Autodesk Fusion 360 part; units mm, degrees
note: some values were not read from the file. Set by a fixed rule: which face or edge a step refers to.
(part 3 of 4)
sketch "Sketch2 (4)" plane through (0, 0, 58.4) normal (0, 0, -1) x (1, 0, 0) in component "M5xxx-lid"
  line L0 (-91.022, 50.6335) -> (-91.022, 57.5617)
  line L1 (-91.022, 57.5617) -> (-97.022, 61.0258)
  line L2 (-97.022, 61.0258) -> (-103.022, 57.5617)
  line L3 (-103.022, 57.5617) -> (-103.022, 50.6335)
  line L4 (-103.022, 50.6335) -> (-97.022, 47.1694)
  line L5 (-97.022, 47.1694) -> (-91.022, 50.6335)
  line L6 (-96.022, 38.6335) -> (-90.022, 35.1694)
  line L7 (-90.022, 35.1694) -> (-84.022, 38.6335)
  line L8 (-96.022, 45.5617) -> (-96.022, 38.6335)
  line L9 (-84.022, 38.6335) -> (-84.022, 45.5617)
  line L10 (-90.022, 49.0258) -> (-96.022, 45.5617)
  line L11 (-84.022, 45.5617) -> (-90.022, 49.0258)
  line L12 (-82.022, 38.6335) -> (-76.022, 35.1694)
  line L13 (-82.022, 45.5617) -> (-82.022, 38.6335)
  line L14 (-70.022, 45.5617) -> (-76.022, 49.0258)
  line L15 (-76.022, 49.0258) -> (-82.022, 45.5617)
  line L16 (-76.022, 35.1694) -> (-70.022, 38.6335)
  line L17 (-83.022, 61.0258) -> (-89.022, 57.5617)
  line L18 (-77.022, 57.5617) -> (-83.022, 61.0258)
  line L19 (-70.022, 38.6335) -> (-70.022, 45.5617)
  line L20 (-83.022, 47.1694) -> (-77.022, 50.6335)
  line L21 (-89.022, 50.6335) -> (-83.022, 47.1694)
  line L22 (-89.022, 57.5617) -> (-89.022, 50.6335)
  line L23 (-77.022, 50.6335) -> (-77.022, 57.5617)
  line L24 (-68.022, 38.6335) -> (-62.022, 35.1694)
  line L25 (-68.022, 45.5617) -> (-68.022, 38.6335)
  line L26 (-56.022, 45.5617) -> (-62.022, 49.0258)
  line L27 (-62.022, 49.0258) -> (-68.022, 45.5617)
  line L28 (-62.022, 35.1694) -> (-56.022, 38.6335)
  line L29 (-69.022, 61.0258) -> (-75.022, 57.5617)
  line L30 (-63.022, 57.5617) -> (-69.022, 61.0258)
  line L31 (-56.022, 38.6335) -> (-56.022, 45.5617)
  line L32 (-69.022, 47.1694) -> (-63.022, 50.6335)
  line L33 (-75.022, 50.6335) -> (-69.022, 47.1694)
  line L34 (-75.022, 57.5617) -> (-75.022, 50.6335)
  line L35 (-63.022, 50.6335) -> (-63.022, 57.5617)
  line L36 (-54.022, 38.6335) -> (-48.022, 35.1694)
  line L37 (-54.022, 45.5617) -> (-54.022, 38.6335)
  line L38 (-42.022, 45.5617) -> (-48.022, 49.0258)
  line L39 (-48.022, 49.0258) -> (-54.022, 45.5617)
  line L40 (-48.022, 35.1694) -> (-42.022, 38.6335)
  line L41 (-55.022, 61.0258) -> (-61.022, 57.5617)
  line L42 (-49.022, 57.5617) -> (-55.022, 61.0258)
  line L43 (-42.022, 38.6335) -> (-42.022, 45.5617)
  line L44 (-55.022, 47.1694) -> (-49.022, 50.6335)
  line L45 (-61.022, 50.6335) -> (-55.022, 47.1694)
  line L46 (-61.022, 57.5617) -> (-61.022, 50.6335)
  line L47 (-49.022, 50.6335) -> (-49.022, 57.5617)
  line L48 (-40.022, 38.6335) -> (-34.022, 35.1694)
  line L49 (-40.022, 45.5617) -> (-40.022, 38.6335)
  line L50 (-28.022, 45.5617) -> (-34.022, 49.0258)
  line L51 (-34.022, 49.0258) -> (-40.022, 45.5617)
  line L52 (-34.022, 35.1694) -> (-28.022, 38.6335)
  line L53 (-41.022, 61.0258) -> (-47.022, 57.5617)
  line L54 (-35.022, 57.5617) -> (-41.022, 61.0258)
  line L55 (-28.022, 38.6335) -> (-28.022, 45.5617)
  line L56 (-41.022, 47.1694) -> (-35.022, 50.6335)
  line L57 (-47.022, 50.6335) -> (-41.022, 47.1694)
  line L58 (-47.022, 57.5617) -> (-47.022, 50.6335)
  line L59 (-35.022, 50.6335) -> (-35.022, 57.5617)
  line L60 (-26.022, 38.6335) -> (-20.022, 35.1694)
  line L61 (-26.022, 45.5617) -> (-26.022, 38.6335)
  line L62 (-14.022, 45.5617) -> (-20.022, 49.0258)
  line L63 (-20.022, 49.0258) -> (-26.022, 45.5617)
  line L64 (-20.022, 35.1694) -> (-14.022, 38.6335)
  line L65 (-27.022, 61.0258) -> (-33.022, 57.5617)
  line L66 (-21.022, 57.5617) -> (-27.022, 61.0258)
  line L67 (-14.022, 38.6335) -> (-14.022, 45.5617)
  line L68 (-27.022, 47.1694) -> (-21.022, 50.6335)
  line L69 (-33.022, 50.6335) -> (-27.022, 47.1694)
  line L70 (-33.022, 57.5617) -> (-33.022, 50.6335)
  line L71 (-21.022, 50.6335) -> (-21.022, 57.5617)
  line L72 (-12.022, 38.6335) -> (-6.022, 35.1694)
  line L73 (-12.022, 45.5617) -> (-12.022, 38.6335)
  line L74 (-0.022, 45.5617) -> (-6.022, 49.0258)
  line L75 (-6.022, 49.0258) -> (-12.022, 45.5617)
  line L76 (-6.022, 35.1694) -> (-0.022, 38.6335)
  line L77 (-13.022, 61.0258) -> (-19.022, 57.5617)
  line L78 (-7.022, 57.5617) -> (-13.022, 61.0258)
  line L79 (-0.022, 38.6335) -> (-0.022, 45.5617)
  line L80 (-13.022, 47.1694) -> (-7.022, 50.6335)
  line L81 (-19.022, 50.6335) -> (-13.022, 47.1694)
  line L82 (-19.022, 57.5617) -> (-19.022, 50.6335)
  line L83 (-7.022, 50.6335) -> (-7.022, 57.5617)
  line L84 (1.978, 38.6335) -> (7.978, 35.1694)
  line L85 (1.978, 45.5617) -> (1.978, 38.6335)
  line L86 (13.978, 45.5617) -> (7.978, 49.0258)
  line L87 (7.978, 49.0258) -> (1.978, 45.5617)
  line L88 (7.978, 35.1694) -> (13.978, 38.6335)
  line L89 (0.978, 61.0258) -> (-5.022, 57.5617)
  line L90 (6.978, 57.5617) -> (0.978, 61.0258)
  line L91 (13.978, 38.6335) -> (13.978, 45.5617)
  line L92 (0.978, 47.1694) -> (6.978, 50.6335)
  line L93 (-5.022, 50.6335) -> (0.978, 47.1694)
  line L94 (-5.022, 57.5617) -> (-5.022, 50.6335)
  line L95 (6.978, 50.6335) -> (6.978, 57.5617)
  line L96 (15.978, 38.6335) -> (21.978, 35.1694)
  line L97 (15.978, 45.5617) -> (15.978, 38.6335)
  line L98 (27.978, 45.5617) -> (21.978, 49.0258)
  line L99 (21.978, 49.0258) -> (15.978, 45.5617)
  line L100 (21.978, 35.1694) -> (27.978, 38.6335)
  line L101 (14.978, 61.0258) -> (8.978, 57.5617)
  line L102 (20.978, 57.5617) -> (14.978, 61.0258)
  line L103 (27.978, 38.6335) -> (27.978, 45.5617)
  line L104 (14.978, 47.1694) -> (20.978, 50.6335)
  line L105 (8.978, 50.6335) -> (14.978, 47.1694)
  line L106 (8.978, 57.5617) -> (8.978, 50.6335)
  line L107 (20.978, 50.6335) -> (20.978, 57.5617)
  line L108 (29.978, 38.6335) -> (35.978, 35.1694)
  line L109 (29.978, 45.5617) -> (29.978, 38.6335)
  line L110 (41.978, 45.5617) -> (35.978, 49.0258)
  line L111 (35.978, 49.0258) -> (29.978, 45.5617)
  line L112 (35.978, 35.1694) -> (41.978, 38.6335)
  line L113 (28.978, 61.0258) -> (22.978, 57.5617)
  line L114 (34.978, 57.5617) -> (28.978, 61.0258)
  line L115 (41.978, 38.6335) -> (41.978, 45.5617)
  line L116 (28.978, 47.1694) -> (34.978, 50.6335)
  line L117 (22.978, 50.6335) -> (28.978, 47.1694)
  line L118 (22.978, 57.5617) -> (22.978, 50.6335)
  line L119 (34.978, 50.6335) -> (34.978, 57.5617)
  line L120 (43.978, 38.6335) -> (49.978, 35.1694)
  line L121 (43.978, 45.5617) -> (43.978, 38.6335)
  line L122 (55.978, 45.5617) -> (49.978, 49.0258)
  line L123 (49.978, 49.0258) -> (43.978, 45.5617)
  line L124 (49.978, 35.1694) -> (55.978, 38.6335)
  line L125 (42.978, 61.0258) -> (36.978, 57.5617)
  line L126 (48.978, 57.5617) -> (42.978, 61.0258)
  line L127 (55.978, 38.6335) -> (55.978, 45.5617)
  line L128 (42.978, 47.1694) -> (48.978, 50.6335)
  line L129 (36.978, 50.6335) -> (42.978, 47.1694)
  line L130 (36.978, 57.5617) -> (36.978, 50.6335)
  line L131 (48.978, 50.6335) -> (48.978, 57.5617)
  line L132 (57.978, 38.6335) -> (63.978, 35.1694)
  line L133 (57.978, 45.5617) -> (57.978, 38.6335)
  line L134 (69.978, 45.5617) -> (63.978, 49.0258)
  line L135 (63.978, 49.0258) -> (57.978, 45.5617)
  line L136 (63.978, 35.1694) -> (69.978, 38.6335)
  line L137 (56.978, 61.0258) -> (50.978, 57.5617)
  line L138 (62.978, 57.5617) -> (56.978, 61.0258)
  line L139 (69.978, 38.6335) -> (69.978, 45.5617)
  line L140 (56.978, 47.1694) -> (62.978, 50.6335)
  line L141 (50.978, 50.6335) -> (56.978, 47.1694)
  line L142 (50.978, 57.5617) -> (50.978, 50.6335)
  line L143 (62.978, 50.6335) -> (62.978, 57.5617)
  line L144 (71.978, 38.6335) -> (77.978, 35.1694)
  line L145 (71.978, 45.5617) -> (71.978, 38.6335)
  line L146 (83.978, 45.5617) -> (77.978, 49.0258)
  line L147 (77.978, 49.0258) -> (71.978, 45.5617)
  line L148 (77.978, 35.1694) -> (83.978, 38.6335)
  line L149 (70.978, 61.0258) -> (64.978, 57.5617)
  line L150 (76.978, 57.5617) -> (70.978, 61.0258)
  line L151 (83.978, 38.6335) -> (83.978, 45.5617)
  line L152 (70.978, 47.1694) -> (76.978, 50.6335)
  line L153 (64.978, 50.6335) -> (70.978, 47.1694)
  line L154 (64.978, 57.5617) -> (64.978, 50.6335)
  line L155 (76.978, 50.6335) -> (76.978, 57.5617)
  line L156 (85.978, 38.6335) -> (91.978, 35.1694)
  line L157 (85.978, 45.5617) -> (85.978, 38.6335)
  line L158 (97.978, 45.5617) -> (91.978, 49.0258)
  line L159 (91.978, 49.0258) -> (85.978, 45.5617)
  line L160 (91.978, 35.1694) -> (97.978, 38.6335)
  line L161 (84.978, 61.0258) -> (78.978, 57.5617)
  line L162 (90.978, 57.5617) -> (84.978, 61.0258)
  line L163 (97.978, 38.6335) -> (97.978, 45.5617)
  line L164 (84.978, 47.1694) -> (90.978, 50.6335)
  line L165 (78.978, 50.6335) -> (84.978, 47.1694)
  line L166 (78.978, 57.5617) -> (78.978, 50.6335)
  line L167 (90.978, 50.6335) -> (90.978, 57.5617)
  line L168 (-96.022, 14.6335) -> (-90.022, 11.1694)
  line L169 (-96.022, 21.5617) -> (-96.022, 14.6335)
  line L170 (-84.022, 21.5617) -> (-90.022, 25.0258)
  line L171 (-90.022, 25.0258) -> (-96.022, 21.5617)
  line L172 (-90.022, 11.1694) -> (-84.022, 14.6335)
  line L173 (-97.022, 37.0258) -> (-103.022, 33.5617)
  line L174 (-91.022, 33.5617) -> (-97.022, 37.0258)
  line L175 (-84.022, 14.6335) -> (-84.022, 21.5617)
  line L176 (-97.022, 23.1694) -> (-91.022, 26.6335)
  line L177 (-103.022, 26.6335) -> (-97.022, 23.1694)
  line L178 (-103.022, 33.5617) -> (-103.022, 26.6335)
  line L179 (-91.022, 26.6335) -> (-91.022, 33.5617)
  line L180 (-82.022, 14.6335) -> (-76.022, 11.1694)
  line L181 (-82.022, 21.5617) -> (-82.022, 14.6335)
  line L182 (-70.022, 21.5617) -> (-76.022, 25.0258)
  line L183 (-76.022, 25.0258) -> (-82.022, 21.5617)
  line L184 (-76.022, 11.1694) -> (-70.022, 14.6335)
  line L185 (-83.022, 37.0258) -> (-89.022, 33.5617)
  line L186 (-77.022, 33.5617) -> (-83.022, 37.0258)
  line L187 (-70.022, 14.6335) -> (-70.022, 21.5617)
  line L188 (-83.022, 23.1694) -> (-77.022, 26.6335)
  line L189 (-89.022, 26.6335) -> (-83.022, 23.1694)
  line L190 (-89.022, 33.5617) -> (-89.022, 26.6335)
  line L191 (-77.022, 26.6335) -> (-77.022, 33.5617)
  line L192 (-68.022, 14.6335) -> (-62.022, 11.1694)
  line L193 (-68.022, 21.5617) -> (-68.022, 14.6335)
  line L194 (-56.022, 21.5617) -> (-62.022, 25.0258)
  line L195 (-62.022, 25.0258) -> (-68.022, 21.5617)
  line L196 (-62.022, 11.1694) -> (-56.022, 14.6335)
  line L197 (-69.022, 37.0258) -> (-75.022, 33.5617)
  line L198 (-63.022, 33.5617) -> (-69.022, 37.0258)
  line L199 (-56.022, 14.6335) -> (-56.022, 21.5617)
  line L200 (-69.022, 23.1694) -> (-63.022, 26.6335)
  line L201 (-75.022, 26.6335) -> (-69.022, 23.1694)
  line L202 (-75.022, 33.5617) -> (-75.022, 26.6335)
  line L203 (-63.022, 26.6335) -> (-63.022, 33.5617)
  line L204 (-54.022, 14.6335) -> (-48.022, 11.1694)
  line L205 (-54.022, 21.5617) -> (-54.022, 14.6335)
  line L206 (-42.022, 21.5617) -> (-48.022, 25.0258)
  line L207 (-48.022, 25.0258) -> (-54.022, 21.5617)
  line L208 (-48.022, 11.1694) -> (-42.022, 14.6335)
  line L209 (-55.022, 37.0258) -> (-61.022, 33.5617)
  line L210 (-49.022, 33.5617) -> (-55.022, 37.0258)
  line L211 (-42.022, 14.6335) -> (-42.022, 21.5617)
  line L212 (-55.022, 23.1694) -> (-49.022, 26.6335)
  line L213 (-61.022, 26.6335) -> (-55.022, 23.1694)
  line L214 (-61.022, 33.5617) -> (-61.022, 26.6335)
  line L215 (-49.022, 26.6335) -> (-49.022, 33.5617)
  line L216 (-40.022, 14.6335) -> (-34.022, 11.1694)
  line L217 (-40.022, 21.5617) -> (-40.022, 14.6335)
  line L218 (-28.022, 21.5617) -> (-34.022, 25.0258)
  line L219 (-34.022, 25.0258) -> (-40.022, 21.5617)
  line L220 (-34.022, 11.1694) -> (-28.022, 14.6335)
  line L221 (-41.022, 37.0258) -> (-47.022, 33.5617)
  line L222 (-35.022, 33.5617) -> (-41.022, 37.0258)
  line L223 (-28.022, 14.6335) -> (-28.022, 21.5617)
  line L224 (-41.022, 23.1694) -> (-35.022, 26.6335)
  line L225 (-47.022, 26.6335) -> (-41.022, 23.1694)
  line L226 (-47.022, 33.5617) -> (-47.022, 26.6335)
  line L227 (-35.022, 26.6335) -> (-35.022, 33.5617)
  line L228 (-26.022, 14.6335) -> (-20.022, 11.1694)
  line L229 (-26.022, 21.5617) -> (-26.022, 14.6335)
  line L230 (-14.022, 21.5617) -> (-20.022, 25.0258)
  line L231 (-20.022, 25.0258) -> (-26.022, 21.5617)
  line L232 (-20.022, 11.1694) -> (-14.022, 14.6335)
  line L233 (-27.022, 37.0258) -> (-33.022, 33.5617)
  line L234 (-21.022, 33.5617) -> (-27.022, 37.0258)
  line L235 (-14.022, 14.6335) -> (-14.022, 21.5617)
  line L236 (-27.022, 23.1694) -> (-21.022, 26.6335)
  line L237 (-33.022, 26.6335) -> (-27.022, 23.1694)
  line L238 (-33.022, 33.5617) -> (-33.022, 26.6335)
  line L239 (-21.022, 26.6335) -> (-21.022, 33.5617)
  line L240 (-12.022, 14.6335) -> (-6.022, 11.1694)
  line L241 (-12.022, 21.5617) -> (-12.022, 14.6335)
  line L242 (-0.022, 21.5617) -> (-6.022, 25.0258)
  line L243 (-6.022, 25.0258) -> (-12.022, 21.5617)
  line L244 (-6.022, 11.1694) -> (-0.022, 14.6335)
  line L245 (-13.022, 37.0258) -> (-19.022, 33.5617)
  line L246 (-7.022, 33.5617) -> (-13.022, 37.0258)
  line L247 (-0.022, 14.6335) -> (-0.022, 21.5617)
  line L248 (-13.022, 23.1694) -> (-7.022, 26.6335)
  line L249 (-19.022, 26.6335) -> (-13.022, 23.1694)
  line L250 (-19.022, 33.5617) -> (-19.022, 26.6335)
  line L251 (-7.022, 26.6335) -> (-7.022, 33.5617)
  line L252 (1.978, 14.6335) -> (7.978, 11.1694)
  line L253 (1.978, 21.5617) -> (1.978, 14.6335)
  line L254 (13.978, 21.5617) -> (7.978, 25.0258)
  line L255 (7.978, 25.0258) -> (1.978, 21.5617)
  line L256 (7.978, 11.1694) -> (13.978, 14.6335)
  line L257 (0.978, 37.0258) -> (-5.022, 33.5617)
  line L258 (6.978, 33.5617) -> (0.978, 37.0258)
  line L259 (13.978, 14.6335) -> (13.978, 21.5617)
  line L260 (0.978, 23.1694) -> (6.978, 26.6335)
  line L261 (-5.022, 26.6335) -> (0.978, 23.1694)
  line L262 (-5.022, 33.5617) -> (-5.022, 26.6335)
  line L263 (6.978, 26.6335) -> (6.978, 33.5617)
  line L264 (15.978, 14.6335) -> (21.978, 11.1694)
  line L265 (15.978, 21.5617) -> (15.978, 14.6335)
  line L266 (27.978, 21.5617) -> (21.978, 25.0258)
  line L267 (21.978, 25.0258) -> (15.978, 21.5617)
  line L268 (21.978, 11.1694) -> (27.978, 14.6335)
  line L269 (14.978, 37.0258) -> (8.978, 33.5617)
  line L270 (20.978, 33.5617) -> (14.978, 37.0258)
  line L271 (27.978, 14.6335) -> (27.978, 21.5617)
  line L272 (14.978, 23.1694) -> (20.978, 26.6335)
  line L273 (8.978, 26.6335) -> (14.978, 23.1694)
  line L274 (8.978, 33.5617) -> (8.978, 26.6335)
  line L275 (20.978, 26.6335) -> (20.978, 33.5617)
  line L276 (29.978, 14.6335) -> (35.978, 11.1694)
  line L277 (29.978, 21.5617) -> (29.978, 14.6335)
  line L278 (41.978, 21.5617) -> (35.978, 25.0258)
  line L279 (35.978, 25.0258) -> (29.978, 21.5617)
  line L280 (35.978, 11.1694) -> (41.978, 14.6335)
  line L281 (28.978, 37.0258) -> (22.978, 33.5617)
  line L282 (34.978, 33.5617) -> (28.978, 37.0258)
  line L283 (41.978, 14.6335) -> (41.978, 21.5617)
  line L284 (28.978, 23.1694) -> (34.978, 26.6335)
  line L285 (22.978, 26.6335) -> (28.978, 23.1694)
  line L286 (22.978, 33.5617) -> (22.978, 26.6335)
  line L287 (34.978, 26.6335) -> (34.978, 33.5617)
  line L288 (43.978, 14.6335) -> (49.978, 11.1694)
  line L289 (43.978, 21.5617) -> (43.978, 14.6335)
  line L290 (55.978, 21.5617) -> (49.978, 25.0258)
  line L291 (49.978, 25.0258) -> (43.978, 21.5617)
  line L292 (49.978, 11.1694) -> (55.978, 14.6335)
  line L293 (42.978, 37.0258) -> (36.978, 33.5617)
  line L294 (48.978, 33.5617) -> (42.978, 37.0258)
  line L295 (55.978, 14.6335) -> (55.978, 21.5617)
  line L296 (42.978, 23.1694) -> (48.978, 26.6335)
  line L297 (36.978, 26.6335) -> (42.978, 23.1694)
  line L298 (36.978, 33.5617) -> (36.978, 26.6335)
  line L299 (48.978, 26.6335) -> (48.978, 33.5617)
  line L300 (57.978, 14.6335) -> (63.978, 11.1694)
  line L301 (57.978, 21.5617) -> (57.978, 14.6335)
  line L302 (69.978, 21.5617) -> (63.978, 25.0258)
  line L303 (63.978, 25.0258) -> (57.978, 21.5617)
  line L304 (63.978, 11.1694) -> (69.978, 14.6335)
  line L305 (56.978, 37.0258) -> (50.978, 33.5617)
  line L306 (62.978, 33.5617) -> (56.978, 37.0258)
  line L307 (69.978, 14.6335) -> (69.978, 21.5617)
  line L308 (56.978, 23.1694) -> (62.978, 26.6335)
  line L309 (50.978, 26.6335) -> (56.978, 23.1694)
  line L310 (50.978, 33.5617) -> (50.978, 26.6335)
  line L311 (62.978, 26.6335) -> (62.978, 33.5617)
  line L312 (71.978, 14.6335) -> (77.978, 11.1694)
  line L313 (71.978, 21.5617) -> (71.978, 14.6335)
  line L314 (83.978, 21.5617) -> (77.978, 25.0258)
  line L315 (77.978, 25.0258) -> (71.978, 21.5617)
  line L316 (77.978, 11.1694) -> (83.978, 14.6335)
  line L317 (70.978, 37.0258) -> (64.978, 33.5617)
  line L318 (76.978, 33.5617) -> (70.978, 37.0258)
  line L319 (83.978, 14.6335) -> (83.978, 21.5617)
  line L320 (70.978, 23.1694) -> (76.978, 26.6335)
  line L321 (64.978, 26.6335) -> (70.978, 23.1694)
  line L322 (64.978, 33.5617) -> (64.978, 26.6335)
  line L323 (76.978, 26.6335) -> (76.978, 33.5617)
  line L324 (85.978, 14.6335) -> (91.978, 11.1694)
  line L325 (85.978, 21.5617) -> (85.978, 14.6335)
  line L326 (97.978, 21.5617) -> (91.978, 25.0258)
  line L327 (91.978, 25.0258) -> (85.978, 21.5617)
  line L328 (91.978, 11.1694) -> (97.978, 14.6335)
  line L329 (84.978, 37.0258) -> (78.978, 33.5617)
  line L330 (90.978, 33.5617) -> (84.978, 37.0258)
  line L331 (97.978, 14.6335) -> (97.978, 21.5617)
  line L332 (84.978, 23.1694) -> (90.978, 26.6335)
  line L333 (78.978, 26.6335) -> (84.978, 23.1694)
  line L334 (78.978, 33.5617) -> (78.978, 26.6335)
  line L335 (90.978, 26.6335) -> (90.978, 33.5617)
  line L336 (-96.022, -9.3665) -> (-90.022, -12.8306)
  line L337 (-96.022, -2.4383) -> (-96.022, -9.3665)
  line L338 (-84.022, -2.4383) -> (-90.022, 1.0258)
  line L339 (-90.022, 1.0258) -> (-96.022, -2.4383)
  line L340 (-90.022, -12.8306) -> (-84.022, -9.3665)
  line L341 (-97.022, 13.0258) -> (-103.022, 9.5617)
  line L342 (-91.022, 9.5617) -> (-97.022, 13.0258)
  line L343 (-84.022, -9.3665) -> (-84.022, -2.4383)
  line L344 (-97.022, -0.8306) -> (-91.022, 2.6335)
  line L345 (-103.022, 2.6335) -> (-97.022, -0.8306)
  line L346 (-103.022, 9.5617) -> (-103.022, 2.6335)
  line L347 (-91.022, 2.6335) -> (-91.022, 9.5617)
  line L348 (-82.022, -9.3665) -> (-76.022, -12.8306)
  line L349 (-82.022, -2.4383) -> (-82.022, -9.3665)
  line L350 (-70.022, -2.4383) -> (-76.022, 1.0258)
  line L351 (-76.022, 1.0258) -> (-82.022, -2.4383)
  line L352 (-76.022, -12.8306) -> (-70.022, -9.3665)
  line L353 (-83.022, 13.0258) -> (-89.022, 9.5617)
  line L354 (-77.022, 9.5617) -> (-83.022, 13.0258)
  line L355 (-70.022, -9.3665) -> (-70.022, -2.4383)
  line L356 (-83.022, -0.8306) -> (-77.022, 2.6335)
  line L357 (-89.022, 2.6335) -> (-83.022, -0.8306)
  line L358 (-89.022, 9.5617) -> (-89.022, 2.6335)
  line L359 (-77.022, 2.6335) -> (-77.022, 9.5617)
  line L360 (-68.022, -9.3665) -> (-62.022, -12.8306)
  line L361 (-68.022, -2.4383) -> (-68.022, -9.3665)
  line L362 (-56.022, -2.4383) -> (-62.022, 1.0258)
  line L363 (-62.022, 1.0258) -> (-68.022, -2.4383)
  line L364 (-62.022, -12.8306) -> (-56.022, -9.3665)
  line L365 (-69.022, 13.0258) -> (-75.022, 9.5617)
  line L366 (-63.022, 9.5617) -> (-69.022, 13.0258)
  line L367 (-56.022, -9.3665) -> (-56.022, -2.4383)
  line L368 (-69.022, -0.8306) -> (-63.022, 2.6335)
  line L369 (-75.022, 2.6335) -> (-69.022, -0.8306)
  line L370 (-75.022, 9.5617) -> (-75.022, 2.6335)
  line L371 (-63.022, 2.6335) -> (-63.022, 9.5617)
  line L372 (-54.022, -9.3665) -> (-48.022, -12.8306)
  line L373 (-54.022, -2.4383) -> (-54.022, -9.3665)
  line L374 (-42.022, -2.4383) -> (-48.022, 1.0258)
  line L375 (-48.022, 1.0258) -> (-54.022, -2.4383)
  line L376 (-48.022, -12.8306) -> (-42.022, -9.3665)
  line L377 (-55.022, 13.0258) -> (-61.022, 9.5617)
  line L378 (-49.022, 9.5617) -> (-55.022, 13.0258)
  line L379 (-42.022, -9.3665) -> (-42.022, -2.4383)
  line L380 (-55.022, -0.8306) -> (-49.022, 2.6335)
  line L381 (-61.022, 2.6335) -> (-55.022, -0.8306)
  line L382 (-61.022, 9.5617) -> (-61.022, 2.6335)
  line L383 (-49.022, 2.6335) -> (-49.022, 9.5617)
  line L384 (-40.022, -9.3665) -> (-34.022, -12.8306)
  line L385 (-40.022, -2.4383) -> (-40.022, -9.3665)
  line L386 (-28.022, -2.4383) -> (-34.022, 1.0258)
  line L387 (-34.022, 1.0258) -> (-40.022, -2.4383)
  line L388 (-34.022, -12.8306) -> (-28.022, -9.3665)
  line L389 (-41.022, 13.0258) -> (-47.022, 9.5617)
  line L390 (-35.022, 9.5617) -> (-41.022, 13.0258)
  line L391 (-28.022, -9.3665) -> (-28.022, -2.4383)
  line L392 (-41.022, -0.8306) -> (-35.022, 2.6335)
  line L393 (-47.022, 2.6335) -> (-41.022, -0.8306)
  line L394 (-47.022, 9.5617) -> (-47.022, 2.6335)
  line L395 (-35.022, 2.6335) -> (-35.022, 9.5617)
  line L396 (-26.022, -9.3665) -> (-20.022, -12.8306)
  line L397 (-26.022, -2.4383) -> (-26.022, -9.3665)
  line L398 (-14.022, -2.4383) -> (-20.022, 1.0258)
  line L399 (-20.022, 1.0258) -> (-26.022, -2.4383)
  line L400 (-20.022, -12.8306) -> (-14.022, -9.3665)
  line L401 (-27.022, 13.0258) -> (-33.022, 9.5617)
  line L402 (-21.022, 9.5617) -> (-27.022, 13.0258)
  line L403 (-14.022, -9.3665) -> (-14.022, -2.4383)
  line L404 (-27.022, -0.8306) -> (-21.022, 2.6335)
  line L405 (-33.022, 2.6335) -> (-27.022, -0.8306)
  line L406 (-33.022, 9.5617) -> (-33.022, 2.6335)
  line L407 (-21.022, 2.6335) -> (-21.022, 9.5617)
  line L408 (-12.022, -9.3665) -> (-6.022, -12.8306)
  line L409 (-12.022, -2.4383) -> (-12.022, -9.3665)
  line L410 (-0.022, -2.4383) -> (-6.022, 1.0258)
  line L411 (-6.022, 1.0258) -> (-12.022, -2.4383)
  line L412 (-6.022, -12.8306) -> (-0.022, -9.3665)
  line L413 (-13.022, 13.0258) -> (-19.022, 9.5617)
  line L414 (-7.022, 9.5617) -> (-13.022, 13.0258)
  line L415 (-0.022, -9.3665) -> (-0.022, -2.4383)
  line L416 (-13.022, -0.8306) -> (-7.022, 2.6335)
  line L417 (-19.022, 2.6335) -> (-13.022, -0.8306)
  line L418 (-19.022, 9.5617) -> (-19.022, 2.6335)
  line L419 (-7.022, 2.6335) -> (-7.022, 9.5617)
  line L420 (1.978, -9.3665) -> (7.978, -12.8306)
  line L421 (1.978, -2.4383) -> (1.978, -9.3665)
  line L422 (13.978, -2.4383) -> (7.978, 1.0258)
  line L423 (7.978, 1.0258) -> (1.978, -2.4383)
  line L424 (7.978, -12.8306) -> (13.978, -9.3665)
  line L425 (0.978, 13.0258) -> (-5.022, 9.5617)
  line L426 (6.978, 9.5617) -> (0.978, 13.0258)
  line L427 (13.978, -9.3665) -> (13.978, -2.4383)
  line L428 (0.978, -0.8306) -> (6.978, 2.6335)
  line L429 (-5.022, 2.6335) -> (0.978, -0.8306)
  line L430 (-5.022, 9.5617) -> (-5.022, 2.6335)
  line L431 (6.978, 2.6335) -> (6.978, 9.5617)
  line L432 (15.978, -9.3665) -> (21.978, -12.8306)
  line L433 (15.978, -2.4383) -> (15.978, -9.3665)
  line L434 (27.978, -2.4383) -> (21.978, 1.0258)
  line L435 (21.978, 1.0258) -> (15.978, -2.4383)
  line L436 (21.978, -12.8306) -> (27.978, -9.3665)
  line L437 (14.978, 13.0258) -> (8.978, 9.5617)
  line L438 (20.978, 9.5617) -> (14.978, 13.0258)
  line L439 (27.978, -9.3665) -> (27.978, -2.4383)
  line L440 (14.978, -0.8306) -> (20.978, 2.6335)
  line L441 (8.978, 2.6335) -> (14.978, -0.8306)
  line L442 (8.978, 9.5617) -> (8.978, 2.6335)
  line L443 (20.978, 2.6335) -> (20.978, 9.5617)
  line L444 (29.978, -9.3665) -> (35.978, -12.8306)
  line L445 (29.978, -2.4383) -> (29.978, -9.3665)
  line L446 (41.978, -2.4383) -> (35.978, 1.0258)
  line L447 (35.978, 1.0258) -> (29.978, -2.4383)
  line L448 (35.978, -12.8306) -> (41.978, -9.3665)
  line L449 (28.978, 13.0258) -> (22.978, 9.5617)
  line L450 (34.978, 9.5617) -> (28.978, 13.0258)
  line L451 (41.978, -9.3665) -> (41.978, -2.4383)
  line L452 (28.978, -0.8306) -> (34.978, 2.6335)
  line L453 (22.978, 2.6335) -> (28.978, -0.8306)
  line L454 (22.978, 9.5617) -> (22.978, 2.6335)
  line L455 (34.978, 2.6335) -> (34.978, 9.5617)
  line L456 (43.978, -9.3665) -> (49.978, -12.8306)
  line L457 (43.978, -2.4383) -> (43.978, -9.3665)
  line L458 (55.978, -2.4383) -> (49.978, 1.0258)
  line L459 (49.978, 1.0258) -> (43.978, -2.4383)
  line L460 (49.978, -12.8306) -> (55.978, -9.3665)
  line L461 (42.978, 13.0258) -> (36.978, 9.5617)
  line L462 (48.978, 9.5617) -> (42.978, 13.0258)
  line L463 (55.978, -9.3665) -> (55.978, -2.4383)
  line L464 (42.978, -0.8306) -> (48.978, 2.6335)
  line L465 (36.978, 2.6335) -> (42.978, -0.8306)
  line L466 (36.978, 9.5617) -> (36.978, 2.6335)
  line L467 (48.978, 2.6335) -> (48.978, 9.5617)
  line L468 (57.978, -9.3665) -> (63.978, -12.8306)
  line L469 (57.978, -2.4383) -> (57.978, -9.3665)
  line L470 (69.978, -2.4383) -> (63.978, 1.0258)
  line L471 (63.978, 1.0258) -> (57.978, -2.4383)
  line L472 (63.978, -12.8306) -> (69.978, -9.3665)
  line L473 (56.978, 13.0258) -> (50.978, 9.5617)
  line L474 (62.978, 9.5617) -> (56.978, 13.0258)
  line L475 (69.978, -9.3665) -> (69.978, -2.4383)
  line L476 (56.978, -0.8306) -> (62.978, 2.6335)
  line L477 (50.978, 2.6335) -> (56.978, -0.8306)
  line L478 (50.978, 9.5617) -> (50.978, 2.6335)
  line L479 (62.978, 2.6335) -> (62.978, 9.5617)
  line L480 (71.978, -9.3665) -> (77.978, -12.8306)
  line L481 (71.978, -2.4383) -> (71.978, -9.3665)
  line L482 (83.978, -2.4383) -> (77.978, 1.0258)
  line L483 (77.978, 1.0258) -> (71.978, -2.4383)
  line L484 (77.978, -12.8306) -> (83.978, -9.3665)
  line L485 (70.978, 13.0258) -> (64.978, 9.5617)
  line L486 (76.978, 9.5617) -> (70.978, 13.0258)
  line L487 (83.978, -9.3665) -> (83.978, -2.4383)
  line L488 (70.978, -0.8306) -> (76.978, 2.6335)
  line L489 (64.978, 2.6335) -> (70.978, -0.8306)
  line L490 (64.978, 9.5617) -> (64.978, 2.6335)
  line L491 (76.978, 2.6335) -> (76.978, 9.5617)
  line L492 (85.978, -9.3665) -> (91.978, -12.8306)
  line L493 (85.978, -2.4383) -> (85.978, -9.3665)
  line L494 (97.978, -2.4383) -> (91.978, 1.0258)
  line L495 (91.978, 1.0258) -> (85.978, -2.4383)
  line L496 (91.978, -12.8306) -> (97.978, -9.3665)
  line L497 (84.978, 13.0258) -> (78.978, 9.5617)
  line L498 (90.978, 9.5617) -> (84.978, 13.0258)
  line L499 (97.978, -9.3665) -> (97.978, -2.4383)
  line L500 (84.978, -0.8306) -> (90.978, 2.6335)
  line L501 (78.978, 2.6335) -> (84.978, -0.8306)
  line L502 (78.978, 9.5617) -> (78.978, 2.6335)
  line L503 (90.978, 2.6335) -> (90.978, 9.5617)
  line L504 (-96.022, -33.3665) -> (-90.022, -36.8306)
  line L505 (-96.022, -26.4383) -> (-96.022, -33.3665)
  line L506 (-84.022, -26.4383) -> (-90.022, -22.9742)
  line L507 (-90.022, -22.9742) -> (-96.022, -26.4383)
  line L508 (-90.022, -36.8306) -> (-84.022, -33.3665)
  line L509 (-97.022, -10.9742) -> (-103.022, -14.4383)
  line L510 (-91.022, -14.4383) -> (-97.022, -10.9742)
  line L511 (-84.022, -33.3665) -> (-84.022, -26.4383)
  line L512 (-97.022, -24.8306) -> (-91.022, -21.3665)
  line L513 (-103.022, -21.3665) -> (-97.022, -24.8306)
  line L514 (-103.022, -14.4383) -> (-103.022, -21.3665)
  line L515 (-91.022, -21.3665) -> (-91.022, -14.4383)
  line L516 (-82.022, -33.3665) -> (-76.022, -36.8306)
  line L517 (-82.022, -26.4383) -> (-82.022, -33.3665)
  line L518 (-70.022, -26.4383) -> (-76.022, -22.9742)
  line L519 (-76.022, -22.9742) -> (-82.022, -26.4383)
  line L520 (-76.022, -36.8306) -> (-70.022, -33.3665)
  line L521 (-83.022, -10.9742) -> (-89.022, -14.4383)
  line L522 (-77.022, -14.4383) -> (-83.022, -10.9742)
  line L523 (-70.022, -33.3665) -> (-70.022, -26.4383)
  line L524 (-83.022, -24.8306) -> (-77.022, -21.3665)
  line L525 (-89.022, -21.3665) -> (-83.022, -24.8306)
  line L526 (-89.022, -14.4383) -> (-89.022, -21.3665)
  line L527 (-77.022, -21.3665) -> (-77.022, -14.4383)
  line L528 (-68.022, -33.3665) -> (-62.022, -36.8306)
  line L529 (-68.022, -26.4383) -> (-68.022, -33.3665)
  line L530 (-56.022, -26.4383) -> (-62.022, -22.9742)
  line L531 (-62.022, -22.9742) -> (-68.022, -26.4383)
  line L532 (-62.022, -36.8306) -> (-56.022, -33.3665)
  line L533 (-69.022, -10.9742) -> (-75.022, -14.4383)
  line L534 (-63.022, -14.4383) -> (-69.022, -10.9742)
  line L535 (-56.022, -33.3665) -> (-56.022, -26.4383)
  line L536 (-69.022, -24.8306) -> (-63.022, -21.3665)
  line L537 (-75.022, -21.3665) -> (-69.022, -24.8306)
  line L538 (-75.022, -14.4383) -> (-75.022, -21.3665)
  line L539 (-63.022, -21.3665) -> (-63.022, -14.4383)
  line L540 (-54.022, -33.3665) -> (-48.022, -36.8306)
  line L541 (-54.022, -26.4383) -> (-54.022, -33.3665)
  line L542 (-42.022, -26.4383) -> (-48.022, -22.9742)
  line L543 (-48.022, -22.9742) -> (-54.022, -26.4383)
  line L544 (-48.022, -36.8306) -> (-42.022, -33.3665)
  line L545 (-55.022, -10.9742) -> (-61.022, -14.4383)
  line L546 (-49.022, -14.4383) -> (-55.022, -10.9742)
  line L547 (-42.022, -33.3665) -> (-42.022, -26.4383)
  line L548 (-55.022, -24.8306) -> (-49.022, -21.3665)
  line L549 (-61.022, -21.3665) -> (-55.022, -24.8306)
  line L550 (-61.022, -14.4383) -> (-61.022, -21.3665)
  line L551 (-49.022, -21.3665) -> (-49.022, -14.4383)
  line L552 (-40.022, -33.3665) -> (-34.022, -36.8306)
  line L553 (-40.022, -26.4383) -> (-40.022, -33.3665)
  line L554 (-28.022, -26.4383) -> (-34.022, -22.9742)
  line L555 (-34.022, -22.9742) -> (-40.022, -26.4383)
  line L556 (-34.022, -36.8306) -> (-28.022, -33.3665)
  line L557 (-41.022, -10.9742) -> (-47.022, -14.4383)
  line L558 (-35.022, -14.4383) -> (-41.022, -10.9742)
  line L559 (-28.022, -33.3665) -> (-28.022, -26.4383)
  line L560 (-41.022, -24.8306) -> (-35.022, -21.3665)
  line L561 (-47.022, -21.3665) -> (-41.022, -24.8306)
  line L562 (-47.022, -14.4383) -> (-47.022, -21.3665)
  line L563 (-35.022, -21.3665) -> (-35.022, -14.4383)
  line L564 (-26.022, -33.3665) -> (-20.022, -36.8306)
  line L565 (-26.022, -26.4383) -> (-26.022, -33.3665)
  line L566 (-14.022, -26.4383) -> (-20.022, -22.9742)
  line L567 (-20.022, -22.9742) -> (-26.022, -26.4383)
  line L568 (-20.022, -36.8306) -> (-14.022, -33.3665)
  line L569 (-27.022, -10.9742) -> (-33.022, -14.4383)
  line L570 (-21.022, -14.4383) -> (-27.022, -10.9742)
  line L571 (-14.022, -33.3665) -> (-14.022, -26.4383)
  line L572 (-27.022, -24.8306) -> (-21.022, -21.3665)
  line L573 (-33.022, -21.3665) -> (-27.022, -24.8306)
  line L574 (-33.022, -14.4383) -> (-33.022, -21.3665)
  line L575 (-21.022, -21.3665) -> (-21.022, -14.4383)
  line L576 (-12.022, -33.3665) -> (-6.022, -36.8306)
  line L577 (-12.022, -26.4383) -> (-12.022, -33.3665)
  line L578 (-0.022, -26.4383) -> (-6.022, -22.9742)
  line L579 (-6.022, -22.9742) -> (-12.022, -26.4383)
  line L580 (-6.022, -36.8306) -> (-0.022, -33.3665)
  line L581 (-13.022, -10.9742) -> (-19.022, -14.4383)
  line L582 (-7.022, -14.4383) -> (-13.022, -10.9742)
  line L583 (-0.022, -33.3665) -> (-0.022, -26.4383)
  line L584 (-13.022, -24.8306) -> (-7.022, -21.3665)
  line L585 (-19.022, -21.3665) -> (-13.022, -24.8306)
  line L586 (-19.022, -14.4383) -> (-19.022, -21.3665)
  line L587 (-7.022, -21.3665) -> (-7.022, -14.4383)
  line L588 (1.978, -33.3665) -> (7.978, -36.8306)
  line L589 (1.978, -26.4383) -> (1.978, -33.3665)
  line L590 (13.978, -26.4383) -> (7.978, -22.9742)
  line L591 (7.978, -22.9742) -> (1.978, -26.4383)
  line L592 (7.978, -36.8306) -> (13.978, -33.3665)
  line L593 (0.978, -10.9742) -> (-5.022, -14.4383)
  line L594 (6.978, -14.4383) -> (0.978, -10.9742)
  line L595 (13.978, -33.3665) -> (13.978, -26.4383)
  line L596 (0.978, -24.8306) -> (6.978, -21.3665)
  line L597 (-5.022, -21.3665) -> (0.978, -24.8306)
  line L598 (-5.022, -14.4383) -> (-5.022, -21.3665)
  line L599 (6.978, -21.3665) -> (6.978, -14.4383)
  line L600 (15.978, -33.3665) -> (21.978, -36.8306)
  line L601 (15.978, -26.4383) -> (15.978, -33.3665)
  line L602 (27.978, -26.4383) -> (21.978, -22.9742)
  line L603 (21.978, -22.9742) -> (15.978, -26.4383)
  line L604 (21.978, -36.8306) -> (27.978, -33.3665)
  line L605 (14.978, -10.9742) -> (8.978, -14.4383)
  line L606 (20.978, -14.4383) -> (14.978, -10.9742)
  line L607 (27.978, -33.3665) -> (27.978, -26.4383)
  line L608 (14.978, -24.8306) -> (20.978, -21.3665)
  line L609 (8.978, -21.3665) -> (14.978, -24.8306)
  line L610 (8.978, -14.4383) -> (8.978, -21.3665)
  line L611 (20.978, -21.3665) -> (20.978, -14.4383)
  line L612 (29.978, -33.3665) -> (35.978, -36.8306)
  line L613 (29.978, -26.4383) -> (29.978, -33.3665)
  line L614 (41.978, -26.4383) -> (35.978, -22.9742)
  line L615 (35.978, -22.9742) -> (29.978, -26.4383)
  line L616 (35.978, -36.8306) -> (41.978, -33.3665)
  line L617 (28.978, -10.9742) -> (22.978, -14.4383)
  line L618 (34.978, -14.4383) -> (28.978, -10.9742)
  line L619 (41.978, -33.3665) -> (41.978, -26.4383)
  line L620 (28.978, -24.8306) -> (34.978, -21.3665)
  line L621 (22.978, -21.3665) -> (28.978, -24.8306)
  line L622 (22.978, -14.4383) -> (22.978, -21.3665)
  line L623 (34.978, -21.3665) -> (34.978, -14.4383)
  line L624 (43.978, -33.3665) -> (49.978, -36.8306)
  line L625 (43.978, -26.4383) -> (43.978, -33.3665)
  line L626 (55.978, -26.4383) -> (49.978, -22.9742)
  line L627 (49.978, -22.9742) -> (43.978, -26.4383)
  line L628 (49.978, -36.8306) -> (55.978, -33.3665)
  line L629 (42.978, -10.9742) -> (36.978, -14.4383)
  line L630 (48.978, -14.4383) -> (42.978, -10.9742)
  line L631 (55.978, -33.3665) -> (55.978, -26.4383)
  line L632 (42.978, -24.8306) -> (48.978, -21.3665)
  line L633 (36.978, -21.3665) -> (42.978, -24.8306)
  line L634 (36.978, -14.4383) -> (36.978, -21.3665)
  line L635 (48.978, -21.3665) -> (48.978, -14.4383)
  line L636 (57.978, -33.3665) -> (63.978, -36.8306)
  line L637 (57.978, -26.4383) -> (57.978, -33.3665)
  line L638 (69.978, -26.4383) -> (63.978, -22.9742)
  line L639 (63.978, -22.9742) -> (57.978, -26.4383)
  line L640 (63.978, -36.8306) -> (69.978, -33.3665)
  line L641 (56.978, -10.9742) -> (50.978, -14.4383)
  line L642 (62.978, -14.4383) -> (56.978, -10.9742)
  line L643 (69.978, -33.3665) -> (69.978, -26.4383)
  line L644 (56.978, -24.8306) -> (62.978, -21.3665)
  line L645 (50.978, -21.3665) -> (56.978, -24.8306)
  line L646 (50.978, -14.4383) -> (50.978, -21.3665)
  line L647 (62.978, -21.3665) -> (62.978, -14.4383)
  line L648 (71.978, -33.3665) -> (77.978, -36.8306)
  line L649 (71.978, -26.4383) -> (71.978, -33.3665)
  line L650 (83.978, -26.4383) -> (77.978, -22.9742)
  line L651 (77.978, -22.9742) -> (71.978, -26.4383)
  line L652 (77.978, -36.8306) -> (83.978, -33.3665)
  line L653 (70.978, -10.9742) -> (64.978, -14.4383)
  line L654 (76.978, -14.4383) -> (70.978, -10.9742)
  line L655 (83.978, -33.3665) -> (83.978, -26.4383)
  line L656 (70.978, -24.8306) -> (76.978, -21.3665)
  line L657 (64.978, -21.3665) -> (70.978, -24.8306)
  line L658 (64.978, -14.4383) -> (64.978, -21.3665)
  line L659 (76.978, -21.3665) -> (76.978, -14.4383)
  line L660 (85.978, -33.3665) -> (91.978, -36.8306)
  line L661 (85.978, -26.4383) -> (85.978, -33.3665)
  line L662 (97.978, -26.4383) -> (91.978, -22.9742)
  line L663 (91.978, -22.9742) -> (85.978, -26.4383)
  line L664 (91.978, -36.8306) -> (97.978, -33.3665)
  line L665 (84.978, -10.9742) -> (78.978, -14.4383)
  line L666 (90.978, -14.4383) -> (84.978, -10.9742)
  line L667 (97.978, -33.3665) -> (97.978, -26.4383)
  line L668 (84.978, -24.8306) -> (90.978, -21.3665)
  line L669 (78.978, -21.3665) -> (84.978, -24.8306)
  line L670 (78.978, -14.4383) -> (78.978, -21.3665)
  line L671 (90.978, -21.3665) -> (90.978, -14.4383)
  line L672 (-96.022, -57.3665) -> (-90.022, -60.8306)
  line L673 (-96.022, -50.4383) -> (-96.022, -57.3665)
  line L674 (-84.022, -50.4383) -> (-90.022, -46.9742)
  line L675 (-90.022, -46.9742) -> (-96.022, -50.4383)
  line L676 (-90.022, -60.8306) -> (-84.022, -57.3665)
  line L677 (-97.022, -34.9742) -> (-103.022, -38.4383)
  line L678 (-91.022, -38.4383) -> (-97.022, -34.9742)
  line L679 (-84.022, -57.3665) -> (-84.022, -50.4383)
  line L680 (-97.022, -48.8306) -> (-91.022, -45.3665)
  line L681 (-103.022, -45.3665) -> (-97.022, -48.8306)
  line L682 (-103.022, -38.4383) -> (-103.022, -45.3665)
  line L683 (-91.022, -45.3665) -> (-91.022, -38.4383)
  line L684 (-82.022, -57.3665) -> (-76.022, -60.8306)
  line L685 (-82.022, -50.4383) -> (-82.022, -57.3665)
  line L686 (-70.022, -50.4383) -> (-76.022, -46.9742)
  line L687 (-76.022, -46.9742) -> (-82.022, -50.4383)
  line L688 (-76.022, -60.8306) -> (-70.022, -57.3665)
  line L689 (-83.022, -34.9742) -> (-89.022, -38.4383)
  line L690 (-77.022, -38.4383) -> (-83.022, -34.9742)
  line L691 (-70.022, -57.3665) -> (-70.022, -50.4383)
  line L692 (-83.022, -48.8306) -> (-77.022, -45.3665)
  line L693 (-89.022, -45.3665) -> (-83.022, -48.8306)
  line L694 (-89.022, -38.4383) -> (-89.022, -45.3665)
  line L695 (-77.022, -45.3665) -> (-77.022, -38.4383)
  line L696 (-68.022, -57.3665) -> (-62.022, -60.8306)
  line L697 (-68.022, -50.4383) -> (-68.022, -57.3665)
  line L698 (-56.022, -50.4383) -> (-62.022, -46.9742)
  line L699 (-62.022, -46.9742) -> (-68.022, -50.4383)
  line L700 (-62.022, -60.8306) -> (-56.022, -57.3665)
  line L701 (-69.022, -34.9742) -> (-75.022, -38.4383)
  line L702 (-63.022, -38.4383) -> (-69.022, -34.9742)
  line L703 (-56.022, -57.3665) -> (-56.022, -50.4383)
  line L704 (-69.022, -48.8306) -> (-63.022, -45.3665)
  line L705 (-75.022, -45.3665) -> (-69.022, -48.8306)
  line L706 (-75.022, -38.4383) -> (-75.022, -45.3665)
  line L707 (-63.022, -45.3665) -> (-63.022, -38.4383)
  line L708 (-54.022, -57.3665) -> (-48.022, -60.8306)
  line L709 (-54.022, -50.4383) -> (-54.022, -57.3665)
  line L710 (-42.022, -50.4383) -> (-48.022, -46.9742)
  line L711 (-48.022, -46.9742) -> (-54.022, -50.4383)
  line L712 (-48.022, -60.8306) -> (-42.022, -57.3665)
  line L713 (-55.022, -34.9742) -> (-61.022, -38.4383)
  line L714 (-49.022, -38.4383) -> (-55.022, -34.9742)
  line L715 (-42.022, -57.3665) -> (-42.022, -50.4383)
  line L716 (-55.022, -48.8306) -> (-49.022, -45.3665)
  line L717 (-61.022, -45.3665) -> (-55.022, -48.8306)
  line L718 (-61.022, -38.4383) -> (-61.022, -45.3665)
  line L719 (-49.022, -45.3665) -> (-49.022, -38.4383)
  line L720 (-40.022, -57.3665) -> (-34.022, -60.8306)
  line L721 (-40.022, -50.4383) -> (-40.022, -57.3665)
  line L722 (-28.022, -50.4383) -> (-34.022, -46.9742)
  line L723 (-34.022, -46.9742) -> (-40.022, -50.4383)
  line L724 (-34.022, -60.8306) -> (-28.022, -57.3665)
  line L725 (-41.022, -34.9742) -> (-47.022, -38.4383)
  line L726 (-35.022, -38.4383) -> (-41.022, -34.9742)
  line L727 (-28.022, -57.3665) -> (-28.022, -50.4383)
  line L728 (-41.022, -48.8306) -> (-35.022, -45.3665)
  line L729 (-47.022, -45.3665) -> (-41.022, -48.8306)
  line L730 (-47.022, -38.4383) -> (-47.022, -45.3665)
  line L731 (-35.022, -45.3665) -> (-35.022, -38.4383)
  line L732 (-26.022, -57.3665) -> (-20.022, -60.8306)
  line L733 (-26.022, -50.4383) -> (-26.022, -57.3665)
  line L734 (-14.022, -50.4383) -> (-20.022, -46.9742)
  line L735 (-20.022, -46.9742) -> (-26.022, -50.4383)
  line L736 (-20.022, -60.8306) -> (-14.022, -57.3665)
  line L737 (-27.022, -34.9742) -> (-33.022, -38.4383)
  line L738 (-21.022, -38.4383) -> (-27.022, -34.9742)
  line L739 (-14.022, -57.3665) -> (-14.022, -50.4383)
  line L740 (-27.022, -48.8306) -> (-21.022, -45.3665)
  line L741 (-33.022, -45.3665) -> (-27.022, -48.8306)
  line L742 (-33.022, -38.4383) -> (-33.022, -45.3665)
  line L743 (-21.022, -45.3665) -> (-21.022, -38.4383)
  line L744 (-12.022, -57.3665) -> (-6.022, -60.8306)
  line L745 (-12.022, -50.4383) -> (-12.022, -57.3665)
  line L746 (-0.022, -50.4383) -> (-6.022, -46.9742)
  line L747 (-6.022, -46.9742) -> (-12.022, -50.4383)
  line L748 (-6.022, -60.8306) -> (-0.022, -57.3665)
  line L749 (-13.022, -34.9742) -> (-19.022, -38.4383)
  line L750 (-7.022, -38.4383) -> (-13.022, -34.9742)
  line L751 (-0.022, -57.3665) -> (-0.022, -50.4383)
  line L752 (-13.022, -48.8306) -> (-7.022, -45.3665)
  line L753 (-19.022, -45.3665) -> (-13.022, -48.8306)
  line L754 (-19.022, -38.4383) -> (-19.022, -45.3665)
  line L755 (-7.022, -45.3665) -> (-7.022, -38.4383)
  line L756 (1.978, -57.3665) -> (7.978, -60.8306)
  line L757 (1.978, -50.4383) -> (1.978, -57.3665)
  line L758 (13.978, -50.4383) -> (7.978, -46.9742)
  line L759 (7.978, -46.9742) -> (1.978, -50.4383)
  line L760 (7.978, -60.8306) -> (13.978, -57.3665)
  line L761 (0.978, -34.9742) -> (-5.022, -38.4383)
  line L762 (6.978, -38.4383) -> (0.978, -34.9742)
  line L763 (13.978, -57.3665) -> (13.978, -50.4383)
  line L764 (0.978, -48.8306) -> (6.978, -45.3665)
  line L765 (-5.022, -45.3665) -> (0.978, -48.8306)
  line L766 (-5.022, -38.4383) -> (-5.022, -45.3665)
  line L767 (6.978, -45.3665) -> (6.978, -38.4383)
  line L768 (15.978, -57.3665) -> (21.978, -60.8306)
  line L769 (15.978, -50.4383) -> (15.978, -57.3665)
  line L770 (27.978, -50.4383) -> (21.978, -46.9742)
  line L771 (21.978, -46.9742) -> (15.978, -50.4383)
  line L772 (21.978, -60.8306) -> (27.978, -57.3665)
  line L773 (14.978, -34.9742) -> (8.978, -38.4383)
  line L774 (20.978, -38.4383) -> (14.978, -34.9742)
  line L775 (27.978, -57.3665) -> (27.978, -50.4383)
  line L776 (14.978, -48.8306) -> (20.978, -45.3665)
  line L777 (8.978, -45.3665) -> (14.978, -48.8306)
  line L778 (8.978, -38.4383) -> (8.978, -45.3665)
  line L779 (20.978, -45.3665) -> (20.978, -38.4383)
  line L780 (29.978, -57.3665) -> (35.978, -60.8306)
  line L781 (29.978, -50.4383) -> (29.978, -57.3665)
  line L782 (41.978, -50.4383) -> (35.978, -46.9742)
  line L783 (35.978, -46.9742) -> (29.978, -50.4383)
  line L784 (35.978, -60.8306) -> (41.978, -57.3665)
  line L785 (28.978, -34.9742) -> (22.978, -38.4383)
  line L786 (34.978, -38.4383) -> (28.978, -34.9742)
  line L787 (41.978, -57.3665) -> (41.978, -50.4383)
  line L788 (28.978, -48.8306) -> (34.978, -45.3665)
  line L789 (22.978, -45.3665) -> (28.978, -48.8306)
  line L790 (22.978, -38.4383) -> (22.978, -45.3665)
  line L791 (34.978, -45.3665) -> (34.978, -38.4383)
  line L792 (43.978, -57.3665) -> (49.978, -60.8306)
  line L793 (43.978, -50.4383) -> (43.978, -57.3665)
  line L794 (55.978, -50.4383) -> (49.978, -46.9742)
  line L795 (49.978, -46.9742) -> (43.978, -50.4383)
  line L796 (49.978, -60.8306) -> (55.978, -57.3665)
  line L797 (42.978, -34.9742) -> (36.978, -38.4383)
  line L798 (48.978, -38.4383) -> (42.978, -34.9742)
  line L799 (55.978, -57.3665) -> (55.978, -50.4383)
  line L800 (42.978, -48.8306) -> (48.978, -45.3665)
  line L801 (36.978, -45.3665) -> (42.978, -48.8306)
  line L802 (36.978, -38.4383) -> (36.978, -45.3665)
  line L803 (48.978, -45.3665) -> (48.978, -38.4383)
  line L804 (57.978, -57.3665) -> (63.978, -60.8306)
  line L805 (57.978, -50.4383) -> (57.978, -57.3665)
  line L806 (69.978, -50.4383) -> (63.978, -46.9742)
  line L807 (63.978, -46.9742) -> (57.978, -50.4383)
  line L808 (63.978, -60.8306) -> (69.978, -57.3665)
  line L809 (56.978, -34.9742) -> (50.978, -38.4383)
  line L810 (62.978, -38.4383) -> (56.978, -34.9742)
  line L811 (69.978, -57.3665) -> (69.978, -50.4383)
  line L812 (56.978, -48.8306) -> (62.978, -45.3665)
  line L813 (50.978, -45.3665) -> (56.978, -48.8306)
  line L814 (50.978, -38.4383) -> (50.978, -45.3665)
  line L815 (62.978, -45.3665) -> (62.978, -38.4383)
  line L816 (71.978, -57.3665) -> (77.978, -60.8306)
  line L817 (71.978, -50.4383) -> (71.978, -57.3665)
  line L818 (83.978, -50.4383) -> (77.978, -46.9742)
  line L819 (77.978, -46.9742) -> (71.978, -50.4383)
  line L820 (77.978, -60.8306) -> (83.978, -57.3665)
  line L821 (70.978, -34.9742) -> (64.978, -38.4383)
  line L822 (76.978, -38.4383) -> (70.978, -34.9742)
  line L823 (83.978, -57.3665) -> (83.978, -50.4383)
  line L824 (70.978, -48.8306) -> (76.978, -45.3665)
  line L825 (64.978, -45.3665) -> (70.978, -48.8306)
  line L826 (64.978, -38.4383) -> (64.978, -45.3665)
  line L827 (76.978, -45.3665) -> (76.978, -38.4383)
  line L828 (85.978, -57.3665) -> (91.978, -60.8306)
  line L829 (85.978, -50.4383) -> (85.978, -57.3665)
  line L830 (97.978, -50.4383) -> (91.978, -46.9742)
  line L831 (91.978, -46.9742) -> (85.978, -50.4383)
  line L832 (91.978, -60.8306) -> (97.978, -57.3665)
  line L833 (84.978, -34.9742) -> (78.978, -38.4383)
  line L834 (90.978, -38.4383) -> (84.978, -34.9742)
  line L835 (97.978, -57.3665) -> (97.978, -50.4383)
  line L836 (84.978, -48.8306) -> (90.978, -45.3665)
  line L837 (78.978, -45.3665) -> (84.978, -48.8306)
  line L838 (78.978, -38.4383) -> (78.978, -45.3665)
  line L839 (90.978, -45.3665) -> (90.978, -38.4383)
  arc A0 (-104.5, 70) -> (-107, 67.5) centre (-104.5, 67.5) ccw
  line L840 (-107, 67.5) -> (-107, -67.5)
  arc A1 (-107, -67.5) -> (-104.5, -70) centre (-104.5, -67.5) ccw
  line L841 (-104.5, -70) -> (102.5, -70)
  arc A2 (102.5, -70) -> (105, -67.5) centre (102.5, -67.5) ccw
  line L842 (105, -67.5) -> (105, 67.5)
  arc A3 (105, 67.5) -> (102.5, 70) centre (102.5, 67.5) ccw
  line L843 (102.5, 70) -> (-104.5, 70)
  arc A4 (114.4, 70) -> (106, 78.4) centre (106, 70) ccw
  line L844 (106, 78.4) -> (-107, 78.4)
  arc A5 (-107, 78.4) -> (-115.3999, 69.9653) centre (-107, 70) ccw
  line L845 (-115.3999, 69.9653) -> (-115.3999, -69.9653)
  arc A6 (-115.3999, -69.9653) -> (-107, -78.4) centre (-107, -70) ccw
  line L846 (-107, -78.4) -> (106, -78.4)
  arc A7 (106, -78.4) -> (114.4, -70) centre (106, -70) ccw
  line L847 (114.4, -70) -> (114.4, 70)
  line L848 (105, -76) -> (-107, -76)
  arc A8 (-113, -70) -> (-107, -76) centre (-107, -70) ccw
  line L849 (-113, -70) -> (-113, 70)
  arc A9 (-107, 76) -> (-113, 70) centre (-107, 70) ccw
  line L850 (-107, 76) -> (105, 76)
  arc A10 (111, 70) -> (105, 76) centre (105, 70) ccw
  line L851 (111, 70) -> (111, -70)
  arc A11 (105, -76) -> (111, -70) centre (105, -70) ccw
  point P0 (-97.022, 54.0976)
  point P1 (-90.022, 42.0976)
  point P2 (-83.022, 54.0976)
  point P3 (-76.022, 42.0976)
  point P4 (-69.022, 54.0976)
  point P5 (-62.022, 42.0976)
  point P6 (-55.022, 54.0976)
  point P7 (-48.022, 42.0976)
  point P8 (-41.022, 54.0976)
  point P9 (-34.022, 42.0976)
  point P10 (-27.022, 54.0976)
  point P11 (-20.022, 42.0976)
  point P12 (-13.022, 54.0976)
  point P13 (-6.022, 42.0976)
  point P14 (0.978, 54.0976)
  point P15 (7.978, 42.0976)
  point P16 (14.978, 54.0976)
  point P17 (21.978, 42.0976)
  point P18 (28.978, 54.0976)
  point P19 (35.978, 42.0976)
  point P20 (42.978, 54.0976)
  point P21 (49.978, 42.0976)
  point P22 (56.978, 54.0976)
  point P23 (63.978, 42.0976)
  point P24 (70.978, 54.0976)
  point P25 (77.978, 42.0976)
  point P26 (84.978, 54.0976)
  point P27 (91.978, 42.0976)
  point P28 (-97.022, 30.0976)
  point P29 (-90.022, 18.0976)
  point P30 (-83.022, 30.0976)
  point P31 (-76.022, 18.0976)
  point P32 (-69.022, 30.0976)
  point P33 (-62.022, 18.0976)
  point P34 (-55.022, 30.0976)
  point P35 (-48.022, 18.0976)
  point P36 (-41.022, 30.0976)
  point P37 (-34.022, 18.0976)
  point P38 (-27.022, 30.0976)
  point P39 (-20.022, 18.0976)
  point P40 (-13.022, 30.0976)
  point P41 (-6.022, 18.0976)
  point P42 (0.978, 30.0976)
  point P43 (7.978, 18.0976)
  point P44 (14.978, 30.0976)
  point P45 (21.978, 18.0976)
  point P46 (28.978, 30.0976)
  point P47 (35.978, 18.0976)
  point P48 (42.978, 30.0976)
  point P49 (49.978, 18.0976)
  point P50 (56.978, 30.0976)
  point P51 (63.978, 18.0976)
  point P52 (70.978, 30.0976)
  point P53 (77.978, 18.0976)
  point P54 (84.978, 30.0976)
  point P55 (91.978, 18.0976)
  point P56 (-97.022, 6.0976)
  point P57 (-90.022, -5.9024)
  point P58 (-83.022, 6.0976)
  point P59 (-76.022, -5.9024)
  point P60 (-69.022, 6.0976)
  point P61 (-62.022, -5.9024)
  point P62 (-55.022, 6.0976)
  point P63 (-48.022, -5.9024)
  point P64 (-41.022, 6.0976)
  point P65 (-34.022, -5.9024)
  point P66 (-27.022, 6.0976)
  point P67 (-20.022, -5.9024)
  point P68 (-13.022, 6.0976)
  point P69 (-6.022, -5.9024)
  point P70 (0.978, 6.0976)
  point P71 (7.978, -5.9024)
  point P72 (14.978, 6.0976)
  point P73 (21.978, -5.9024)
  point P74 (28.978, 6.0976)
  point P75 (35.978, -5.9024)
  point P76 (42.978, 6.0976)
  point P77 (49.978, -5.9024)
  point P78 (56.978, 6.0976)
  point P79 (63.978, -5.9024)
  point P80 (70.978, 6.0976)
  point P81 (77.978, -5.9024)
  point P82 (84.978, 6.0976)
  point P83 (91.978, -5.9024)
  point P84 (-97.022, -17.9024)
  point P85 (-90.022, -29.9024)
  point P86 (-83.022, -17.9024)
  point P87 (-76.022, -29.9024)
  point P88 (-69.022, -17.9024)
  point P89 (-62.022, -29.9024)
  point P90 (-55.022, -17.9024)
  point P91 (-48.022, -29.9024)
  point P92 (-41.022, -17.9024)
  point P93 (-34.022, -29.9024)
  point P94 (-27.022, -17.9024)
  point P95 (-20.022, -29.9024)
  point P96 (-13.022, -17.9024)
  point P97 (-6.022, -29.9024)
  point P98 (0.978, -17.9024)
  point P99 (7.978, -29.9024)
  point P100 (14.978, -17.9024)
  point P101 (21.978, -29.9024)
  point P102 (28.978, -17.9024)
  point P103 (35.978, -29.9024)
  point P104 (42.978, -17.9024)
  point P105 (49.978, -29.9024)
  point P106 (56.978, -17.9024)
  point P107 (63.978, -29.9024)
  point P108 (70.978, -17.9024)
  point P109 (77.978, -29.9024)
  point P110 (84.978, -17.9024)
  point P111 (91.978, -29.9024)
  point P112 (-97.022, -41.9024)
  point P113 (-90.022, -53.9024)
  point P114 (-83.022, -41.9024)
  point P115 (-76.022, -53.9024)
  point P116 (-69.022, -41.9024)
  point P117 (-62.022, -53.9024)
  point P118 (-55.022, -41.9024)
  point P119 (-48.022, -53.9024)
  point P120 (-41.022, -41.9024)
  point P121 (-34.022, -53.9024)
  point P122 (-27.022, -41.9024)
  point P123 (-20.022, -53.9024)
  point P124 (-13.022, -41.9024)
  point P125 (-6.022, -53.9024)
  point P126 (0.978, -41.9024)
  point P127 (7.978, -53.9024)
  point P128 (14.978, -41.9024)
  point P129 (21.978, -53.9024)
  point P130 (28.978, -41.9024)
  point P131 (35.978, -53.9024)
  point P132 (42.978, -41.9024)
  point P133 (49.978, -53.9024)
  point P134 (56.978, -41.9024)
  point P135 (63.978, -53.9024)
  point P136 (70.978, -41.9024)
  point P137 (77.978, -53.9024)
  point P138 (84.978, -41.9024)
  point P139 (91.978, -53.9024)
  dimension "d258" = 6
  dimension "d259" = 6
  dimension "d262" = 14
  dimension "d263" = -24
  constraint vertical L3
  constraint vertical L8